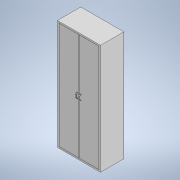
# Autodesk Inventor part: Tablero Eléctrico
Saved by Autodesk Inventor 2020 (Build 240168000, 168)
## iProperties
Created: 2019-10-05
Part Number: Tablero Eléctrico
Material: Genérico
Document SubType Name: Modeling
Designer: dasa1
Density: 1 g/cm^3
Appearance: Valor por defecto
Author: dasa1
Autodesk Inventor part; units mm, degrees
ref_plane "YZ Plane" through (0, 0, 0) normal (1, 0, 0) x (0, 1, 0)
ref_plane "XZ Plane" through (0, 0, 0) normal (0, 1, 0) x (-1, 0, 0)
ref_plane "XY Plane" through (0, 0, 0) normal (0, 0, 1) x (1, 0, 0)
sketch "Boceto1" plane through (0, 0, 0) normal (0, 1, 0) x (-1, 0, 0)
  line L0 (0, 0) -> (-830, 0)
  line L1 (-830, 0) -> (-830, -450)
  line L2 (-830, -450) -> (0, -450)
  line L3 (0, -450) -> (0, 0)
  dimension "d0" = 830
  dimension "d1" = 450
  constraints: 8 end point, 2 parallel, 1 horizontal, 1 perpendicular
  measures "d0" distance of L2.end L1.end
  measures "d1" distance of L1.end L0.end
extrude "Extrusión1" add sketch "Boceto1" along normal blind 2120
sketch "Boceto2" plane through (0, 0, 0) normal (0, 0, 1) x (1, 0, 0)
  line L0 (0, 0) -> (830, 0) construction
  line L1 (830, 0) -> (830, 2120) construction
  line L2 (0, 2120) -> (830, 2120) construction
  line L3 (0, 0) -> (0, 2120) construction
  line L4 (0, 2120) -> (830, 2120) construction
  line L5 (0, 2120) -> (30, 2120) construction
  line L6 (30, 2120) -> (30, 2090) construction
  line L7 (30, 2090) -> (0, 2090) construction
  line L8 (0, 2090) -> (0, 2120) construction
  line L9 (830, 0) -> (830, 2120) construction
  line L10 (830, 0) -> (800, 0) construction
  line L11 (800, 0) -> (800, 30) construction
  line L12 (800, 30) -> (830, 30) construction
  line L13 (830, 30) -> (830, 0) construction
  line L14 (30, 2090) -> (800, 2090)
  line L15 (800, 2090) -> (800, 30)
  line L16 (800, 30) -> (30, 30)
  line L17 (30, 30) -> (30, 2090)
  line L18 (30, 2090) -> (31, 2090) construction
  line L19 (31, 2090) -> (31, 2089) construction
  line L20 (31, 2089) -> (30, 2089) construction
  line L21 (30, 2089) -> (30, 2090) construction
  line L22 (800, 30) -> (799, 30) construction
  line L23 (799, 30) -> (799, 31) construction
  line L24 (799, 31) -> (800, 31) construction
  line L25 (800, 31) -> (800, 30) construction
  line L26 (800, 30) -> (415, 30) construction
  line L27 (415, 30) -> (415.5, 30) construction
  line L28 (415.5, 30) -> (414.5, 30) construction
  line L29 (414.5, 30) -> (414.5, 31) construction
  line L30 (414.5, 31) -> (415.5, 31) construction
  line L31 (415.5, 31) -> (415.5, 30) construction
  line L32 (415.5, 30) -> (415.5, 2090) construction
  line L33 (415.5, 30) -> (2475.5, 30) construction
  line L34 (415.5, 2090) -> (414.5, 2090) construction
  line L35 (414.5, 2090) -> (414.5, 2089) construction
  line L36 (414.5, 2089) -> (415.5, 2089) construction
  line L37 (415.5, 2089) -> (415.5, 2090) construction
  line L38 (415.5, 2089) -> (799, 2089)
  line L39 (799, 2089) -> (799, 31)
  line L40 (799, 31) -> (415.5, 31)
  line L41 (415.5, 31) -> (415.5, 2089)
  line L42 (31, 2089) -> (414.5, 2089)
  line L43 (414.5, 2089) -> (414.5, 31)
  line L44 (414.5, 31) -> (31, 31)
  line L45 (31, 31) -> (31, 2089)
  dimension "d4" = 30
  dimension "d5" = 30
  dimension "d6" = 30
  dimension "d7" = 30
  dimension "d8" = 1
  dimension "d9" = 1
  dimension "d10" = 1
  dimension "d11" = 1
  dimension "d12" = 0.5
  dimension "d13" = 1
  dimension "d14" = 1
  dimension "d15" = 90
  dimension "d16" = 1
  dimension "d17" = 1
  constraints: 80 end point, 18 parallel, 10 horizontal, 10 perpendicular, 2 point on line, 1 midpoint
  measures "d4" distance of L6.end L7.end
  measures "d5" distance of L5.end L6.end
  measures "d6" distance of L11.end L12.end
  measures "d7" distance of L10.end L11.end
  measures "d8" distance of L19.end L20.end
  measures "d9" distance of L18.end L19.end
  measures "d10" distance of L23.end L24.end
  measures "d11" distance of L22.end L23.end
  measures "d12" distance of L26.end L27.end
  measures "d13" distance of L29.end L30.end
  measures "d14" distance of L28.end L29.end
  measures "d15" angle of L33 L32
  measures "d16" distance of L36.end L35.end
  measures "d17" distance of L35.end L34.end
extrude "Extrusión2" cut sketch "Boceto2" against normal blind 10
sketch "Boceto3" plane through (31, 2089, 0) normal (0, 0, 1) x (1, 0, 0)
  line L0 (383.5, 0) -> (0, 0) construction
  line L1 (0, 0) -> (0, -2058) construction
  line L2 (0, -2058) -> (383.5, -2058) construction
  line L3 (383.5, -2058) -> (383.5, 0) construction
  line L4 (768, -2058) -> (768, 0) construction
  line L5 (768, 0) -> (384.5, 0) construction
  line L6 (384.5, 0) -> (384.5, -2058) construction
  line L7 (384.5, -2058) -> (768, -2058) construction
  line L8 (383.5, -2058) -> (383.5, 0) construction
  line L9 (383.5, 0) -> (383.5, -2058) construction
  line L10 (383.5, 0) -> (0, 0) construction
  line L11 (383.5, 0) -> (383.5, -1026) construction
  line L12 (383.5, -1026) -> (363.5, -1026) construction
  line L13 (383.5, -1026) -> (384.5, -1026) construction
  line L14 (384.5, 0) -> (384.5, -2058) construction
  line L15 (384.5, -1026) -> (404.5, -1026) construction
  line L16 (404.5, -1026) -> (404.5, -976) construction
  line L17 (363.5, -1026) -> (363.5, -1076) construction
  line L18 (363.5, -1076) -> (343.5, -1076)
  line L19 (343.5, -1076) -> (343.5, -976)
  line L20 (343.5, -976) -> (363.5, -976)
  line L21 (363.5, -976) -> (363.5, -1076)
  line L22 (404.5, -976) -> (424.5, -976)
  line L23 (424.5, -976) -> (424.5, -1076)
  line L24 (424.5, -1076) -> (404.5, -1076)
  line L25 (404.5, -1076) -> (404.5, -976)
  point P0 (-31, -2089)
  dimension "d21" = 1026
  dimension "d22" = 20
  dimension "d23" = 20
  dimension "d24" = 50
  dimension "d25" = 50
  dimension "d26" = 20
  dimension "d27" = 100
  dimension "d28" = 20
  dimension "d29" = 100
  constraints: 30 end point, 4 parallel, 4 perpendicular, 3 point on line, 3 vertical, 2 horizontal
  measures "d21" distance of L0.start L11.end
  measures "d22" distance of L11.end L12.end
  measures "d23" distance of L13.end L15.end
  measures "d24" distance of L15.end L16.end
  measures "d25" distance of L12.end L17.end
  measures "d26" distance of L19.end L20.end
  measures "d27" distance of L18.end L19.end
  measures "d28" distance of L23.end L24.end
  measures "d29" distance of L22.end L23.end
extrude "Extrusión3" add sketch "Boceto3" along normal blind 25
draft "Cara para el ángulo de desmoldeo1" angle 15 pull direction (0, 0, 1) faces at (387.8333, 1113, 8.3333) fixed edges at (384.5, 1113, 0)
draft "Cara para el ángulo de desmoldeo2" angle 15 pull direction (0, 0, 1) faces at (381.1667, 1013, 8.3333) fixed edges at (384.5, 1013, 0)
draft "Cara para el ángulo de desmoldeo3" angle 15 pull direction (0, 0, 1) fixed plane through (684.5, 1044.3333, 0) normal (0, 0, 1) faces at (442.1667, 1013, 8.3333)
draft "Cara para el ángulo de desmoldeo4" angle 15 pull direction (0, 0, 1) fixed plane through (684.5, 1044.3333, 0) normal (0, 0, 1) faces at (448.8333, 1113, 8.3333)
fillet "Empalme1" radius 20 4 edges at (445.5, 1106.3013, 25) (384.5, 1106.3013, 25) (445.5, 1019.6987, 25) (384.5, 1019.6987, 25)
sketch "Boceto4" plane through (374.5, 1013, 0) normal (-1, 0, 0) x (0, 0, 1)
  arc A0 (10.1764, 2.7268) -> (25, 22.0453) centre (5, 22.0453) ccw projected
  line L0 (25, 77.9547) -> (25, 22.0453) projected
  arc A1 (25, 77.9547) -> (10.1764, 97.2732) centre (5, 77.9547) ccw projected
  line L1 (0, 100) -> (10.1764, 97.2732) projected
  line L2 (0, 0) -> (0, 100) projected
  line L3 (0, 0) -> (10.1764, 2.7268) projected
  arc A2 (22, 77.9547) -> (9.3999, 94.3755) centre (5, 77.9547) ccw
  line L4 (22, 77.9547) -> (22, 22.0453)
  arc A3 (9.3999, 5.6245) -> (22, 22.0453) centre (5, 22.0453) ccw
  line L5 (9.3999, 5.6245) -> (3, 3.9097)
  line L6 (3, 3.9097) -> (3, 96.0903) construction
  line L7 (3, 96.0903) -> (9.3999, 94.3755)
  line L8 (9.3999, 94.3755) -> (0, 96.8942)
  line L9 (0, 100) -> (0, 0) projected
  line L10 (9.3999, 5.6245) -> (0, 3.1058)
  point P0 (0, -1013)
  point P1 (3, 3.9097)
  dimension "d37" = 3
  constraints: 12 end point, 4 point on circle, 2 centre point, 2 point on line, 2 tangent, 5 other
  measures "d37" radial gap between concentric circles of A1 A2
extrude "Extrusión5" cut sketch "Boceto4" against normal blind 81 contours L2 L8 L7 A2 L4 A3 L5 L10
